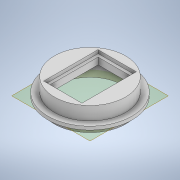
# Autodesk Inventor part: Upper Coll r2ar
Saved by Autodesk Inventor 2020 (Build 240168000, 168)
## iProperties
Created: 2023-10-18
Part Number: Upper Coll r2ar
Material: Generic
Document SubType Name: Modeling
Designer: Beaucage
Density: 1 g/cm^3
Appearance: Default
Author: Beaucage
Autodesk Inventor part; units mm, degrees
ref_plane "YZ Plane" through (0, 0, 0) normal (1, 0, 0) x (0, 1, 0)
ref_plane "XZ Plane" through (0, 0, 0) normal (0, 1, 0) x (-1, 0, 0)
ref_plane "XY Plane" through (0, 0, 0) normal (0, 0, 1) x (1, 0, 0)
sketch "Sketch1" plane through (0, 0, 0) normal (0, 1, 0) x (-1, 0, 0)
  circle A0 centre (0, 0) radius 33.655
  circle A1 centre (0, 0) radius 30.48
  dimension "d0" = 67.31
  dimension "d1" = 60.96
  constraints: 2 centre point, 2 coincident
  measures "d0" diameter of A0
  measures "d1" diameter of A1
extrude "Extrusion1" add sketch "Sketch1" along normal blind 12.7
sketch "Sketch2" plane through (0, 12.7, 0) normal (0, 1, 0) x (1, 0, 0)
  circle A0 centre (0, 0) radius 33.655
  constraints: 1 centre point, 1 coincident
extrude "Extrusion2" add sketch "Sketch2" along normal blind 9.525
sketch "Sketch3" plane through (0, 22.225, 0) normal (0, 1, 0) x (1, 0, 0)
  line L0 (18.0975, -25.7175) -> (-18.0975, -25.7175)
  line L1 (-18.0975, -25.7175) -> (-18.0975, 25.7175)
  line L2 (-18.0975, 25.7175) -> (18.0975, 25.7175)
  line L3 (18.0975, 25.7175) -> (18.0975, -25.7175)
  line L4 (18.0975, -25.7175) -> (-18.0975, 25.7175) construction
  line L5 (-18.0975, -25.7175) -> (18.0975, 25.7175) construction
  point P0 (0, 0)
  dimension "d6" = 36.195
  dimension "d7" = 51.435
  constraints: 12 end point, 2 midpoint, 2 parallel, 1 horizontal, 1 perpendicular
  measures "d6" distance of L1.end L2.end
  measures "d7" distance of L0.end L1.end
extrude "Extrusion3" cut sketch "Sketch3" against normal blind 3.175
sketch "Sketch4" plane through (0, 19.05, 0) normal (0, 1, 0) x (1, 0, 0)
  line L0 (15.24, -22.86) -> (-15.24, -22.86)
  line L1 (-15.24, -22.86) -> (-15.24, 22.86)
  line L2 (-15.24, 22.86) -> (15.24, 22.86)
  line L3 (15.24, 22.86) -> (15.24, -22.86)
  line L4 (15.24, -22.86) -> (-15.24, 22.86) construction
  line L5 (-15.24, -22.86) -> (15.24, 22.86) construction
  point P0 (0, 0)
  dimension "d10" = 30.48
  dimension "d11" = 45.72
  constraints: 12 end point, 2 midpoint, 2 parallel, 1 horizontal, 1 perpendicular
  measures "d10" distance of L1.end L2.end
  measures "d11" distance of L0.end L1.end
extrude "Extrusion4" cut sketch "Sketch4" against normal through all
ref_plane "Work Plane1" through (0, 6.35, 0) normal (0, -1, 0) x (1, 0, 0)
sketch "Sketch5" plane through (0, 6.35, 0) normal (0, -1, 0) x (1, 0, 0)
  circle A0 centre (0, 0) radius 33.655
  circle A1 centre (0, 0) radius 29.8345
  circle A2 centre (0, 0) radius 39.6875
  dimension "d15" = 79.375
  constraints: 3 centre point, 3 coincident
  measures "d15" diameter of A2
extrude "Extrusion5" add sketch "Sketch5" against normal blind 3.175 contours A2
body "Solid1"
